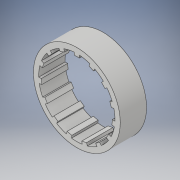
# Autodesk Inventor part: AWAutomobloxTire
Saved by Autodesk Inventor 2018 (Build 220112000, 112)
## iProperties
Created: 2019-01-17
Part Number: AWAutomobloxTire
Material: Generic
Document SubType Name: Modeling
Designer: This kid
Density: 1 g/cm^3
Appearance: Default
Author: This kid
Autodesk Inventor part; units mm, degrees
ref_plane "YZ Plane" through (0, 0, 0) normal (1, 0, 0) x (0, 1, 0)
ref_plane "XZ Plane" through (0, 0, 0) normal (0, 1, 0) x (-1, 0, 0)
ref_plane "XY Plane" through (0, 0, 0) normal (0, 0, 1) x (1, 0, 0)
sketch "Sketch1" plane through (0, 0, 0) normal (0, 0, 1) x (1, 0, 0)
  circle A0 centre (0, 0) radius 20.955
  circle A1 centre (0, 0) radius 18.415
  arc A2 (1.196, 17.1032) -> (-1.196, 17.1032) centre (0, 0) ccw
  line L0 (0, 0) -> (0, 27.5348)
  line L1 (1.196, 17.1032) -> (1.2846, 18.3701)
  line L2 (-1.196, 17.1032) -> (-1.2846, 18.3701)
  dimension "d0" = 41.91
  dimension "d2" = 1.27
  dimension "d3" = 2.54
  constraints: 6 end point, 4 point on circle, 3 centre point, 3 coincident, 1 vertical
  measures "d0" diameter of A0
  measures "d2" radial gap between concentric circles of A2 A1
  measures "d3" radial gap between concentric circles of A1 A0
extrude "Extrusion1" add sketch "Sketch1" along normal blind 12.7
extrude "Extrusion2" add sketch "Sketch1" along normal blind 12.7 contours L1 A2 L0 A1 | A1 L0 A2 L2
pattern_circular "Circular Pattern1" count 15 over 360 about axis through (0, 0, 0) along (0, 0, 1) of "Extrusion2", "Extrusion1"
body "Solid1"
